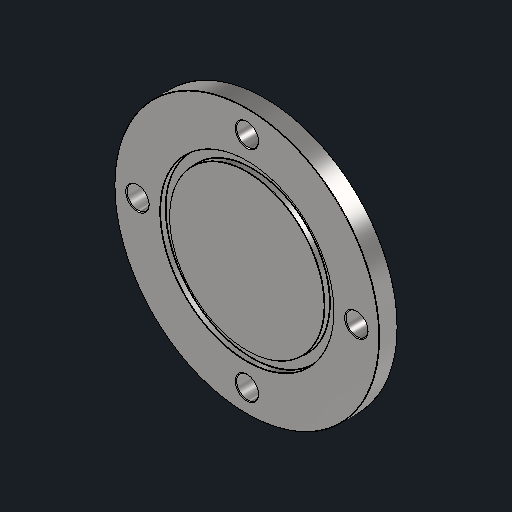
# Autodesk Inventor part: JIS-VG65
Saved by Autodesk Inventor 2026 (Build 300175050, 175E)
## iProperties
Created: 2026-01-06
Part Number: JIS-VG65
Material: Stainless Steel
Document SubType Name: Modeling
Designer: queezz
Density: 8 g/cm^3
Appearance: Semi-Polished
Author: queezz
Autodesk Inventor part; units mm, degrees
ref_plane "YZ Plane" through (0, 0, 0) normal (1, 0, 0) x (0, 1, 0)
ref_plane "XZ Plane" through (0, 0, 0) normal (0, 1, 0) x (-1, 0, 0)
ref_plane "XY Plane" through (0, 0, 0) normal (0, 0, 1) x (1, 0, 0)
sketch "Sketch1" plane through (0, 0, 0) normal (0, 0, 1) x (1, 0, 0)
  circle A0 centre (0, 0) radius 72.5
  dimension "d0" = 145
  constraints: 1 centre point, 1 coincident
  measures "d0" diameter of A0
extrude "Extrusion1" add sketch "Sketch1" along normal blind 10
sketch "Sketch2" plane through (0, 0, 10) normal (0, 0, 1) x (1, 0, 0)
  circle A0 centre (0, 0) radius 60 construction
  point P0 (60, 0)
  dimension "d3" = 120
  constraints: 2 horizontal alignment, 1 coincident, 2 other
hole "Hole1" at (60, 0, 10) direction (0, 0, -1) diameter 12 end through all
pattern_circular "Circular Pattern1" count 4 over 360 about axis through (0, 0, 0) along (0, 0, 1) of "Hole1"
sketch "Sketch3" plane through (0, 0, 10) normal (0, 0, 1) x (1, 0, 0)
  circle A0 centre (0, 0) radius 42.5
  circle A1 centre (0, 0) radius 47.5
  dimension "d14" = 85
  dimension "d15" = 95
  constraints: 2 centre point, 2 coincident
  measures "d14" diameter of A0
  measures "d15" diameter of A1
extrude "Extrusion2" cut sketch "Sketch3" against normal blind 3
fillet "Fillet1" radius 0.2 6 edges at (-72.5, 0, 10) (-72.5, 0, 0) (-47.5, 0, 10) (-42.5, 0, 10) (-47.5, 0, 7) (-42.5, 0, 7)
chamfer "Chamfer1" distance 0.4 angle 45 8 edges at (60, 6, 10) (-6, 60, 10) (-60, -6, 10) (6, -60, 10) (6, -60, 0) (60, 6, 0) (-60, -6, 0) (-6, 60, 0)
body "Solid1"
